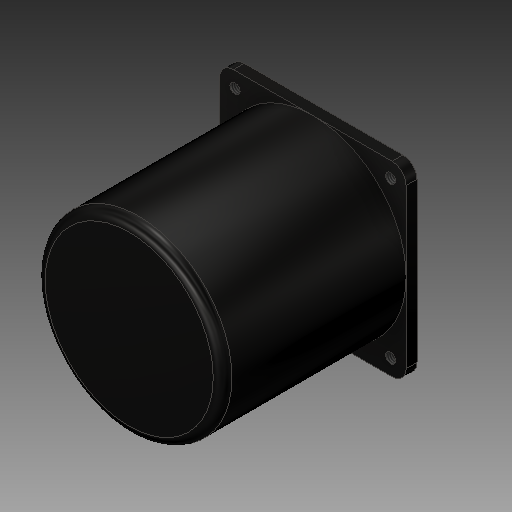
# Autodesk Inventor part: Moteur
Saved by Autodesk Inventor 2017 (Build 210142000, 142)
## iProperties
Company: FABLAB Frenchmakers
Part Number: Moteur
Project: 1400-PopCorn Machine
Material: Acier inoxydable
Catalog Web Link: http://www.frenchmakers.com/
Document SubType Name: Modeling
Designer: FABLAB Frenchmakers
Density: 8 g/cm^3
Appearance: Semi-poli
Stock Number: 1400-07-01
Mass: 1436.32 g
Surface Area: 193.93 cm^2
Volume: 179.539 cm^3
Author: Adrien MARY
Autodesk Inventor part; units mm, degrees
ref_plane "YZ Plane" through (0, 0, 0) normal (1, 0, 0) x (0, 1, 0)
ref_plane "XZ Plane" through (0, 0, 0) normal (0, 1, 0) x (-1, 0, 0)
ref_plane "XY Plane" through (0, 0, 0) normal (0, 0, 1) x (1, 0, 0)
sketch "Esquisse1" plane through (0, 0, 0) normal (0, 0, 1) x (1, 0, 0)
  line L0 (-25.5, -30) -> (25.5, -30)
  line L1 (30, -25.5) -> (30, 25.5)
  line L2 (25.5, 30) -> (-25.5, 30)
  line L3 (-30, 25.5) -> (-30, -25.5)
  line L4 (-30, -30) -> (30, 30) construction
  line L5 (30, -30) -> (-30, 30) construction
  arc A0 (-30, -25.5) -> (-25.5, -30) centre (-25.5, -25.5) ccw
  arc A1 (25.5, -30) -> (30, -25.5) centre (25.5, -25.5) ccw
  arc A2 (30, 25.5) -> (25.5, 30) centre (25.5, 25.5) ccw
  arc A3 (-25.5, 30) -> (-30, 25.5) centre (-25.5, 25.5) ccw
  point P0 (0, 0)
  dimension "d0" = 60
  dimension "d1" = 60
  dimension "d2" = 4.5
  constraints: 12 end point, 8 point on circle, 8 point on line, 8 tangent, 4 centre point, 3 equal radius, 2 midpoint, 2 parallel, 1 horizontal, 1 perpendicular
  measures "d0" distance of L5.end L4.end
  measures "d1" distance of L4.end L5.start
  measures "d2" radius of A0
extrude "Embase" add sketch "Esquisse1" along normal blind 3.5
sketch "Esquisse3" plane through (0, 0, 3.5) normal (0, 0, 1) x (1, 0, 0)
  point P0 (0, 0)
  point P1 (-25, -25)
  point P2 (-25, 25)
  point P3 (25, 25)
  point P4 (25, -25)
  dimension "Entraxe_moteur" = 50
  dimension "d8" = 50
  dimension "d9" = 25
  dimension "d10" = 25
  constraints: 2 horizontal alignment, 2 vertical alignment
  measures "Entraxe_moteur" distance of point (-25, 25) point (25, 25)
  measures "d8" distance of point (25, 25) point (25, -25)
  measures "d9" horizontal distance of point (25, 25) point (0, 0)
  measures "d10" horizontal distance of point (0, 0) point (25, 25)
hole "Perçage1" at (-25, -25, 3.5) at (-25, 25, 3.5) at (25, 25, 3.5) at (25, -25, 3.5) direction (0, 0, -1) diameter 3.242 end through all thread size "M4x0.7" class "6H" standard "ISO Metric profile"
sketch "Esquisse2" plane through (0, 0, 3.5) normal (0, 0, 1) x (1, 0, 0)
  circle A0 centre (0, 0) radius 30
  line L0 (-30, 25.5) -> (-30, -25.5) projected
  constraints: 1 centre point, 1 coincident, 1 tangent
extrude "Extrusion2" add sketch "Esquisse2" along normal blind 59
fillet "Congé1" radius 3 1 edges at (-30, 0, 62.5)
sketch "Esquisse4" plane through (0, 0, 0) normal (0, 0, -1) x (-1, 0, 0)
  circle A0 centre (0, 0) radius 3.5
  dimension "d19" = 7
  constraints: 1 centre point, 1 coincident
  measures "d19" diameter of A0
extrude "Extrusion3" add sketch "Esquisse4" along normal blind 19
sketch "Esquisse5" plane through (0, 0, -19) normal (0, 0, -1) x (-1, 0, 0)
  line L0 (-1.8028, -3) -> (1.8028, -3)
  circle A0 centre (0, 0) radius 3.5 projected
  dimension "d22" = 6.5
  constraints: 2 end point, 2 point on circle, 1 horizontal
extrude "Extrusion4" cut sketch "Esquisse5" against normal blind 15 contours L0 A0 picked at (0.3722, -3.1057)
sketch "Esquisse6" plane through (-1.8028, -3, -19) normal (0, -1, 0) x (1, 0, 0)
  line L0 (3.6056, 0) -> (0, 0) projected
  point P0 (1.8028, 19)
  point P1 (1.8028, 8)
  point P2 (1.8028, 0)
  dimension "d25" = 8
  constraints: 1 midpoint, 1 vertical alignment
  measures "d25" distance from line of L0 point (1.803, 8)
hole "Perçage2" at (0, -3, -11) direction (0, 1, 0) diameter 3.4 end through all clearance for "Vis à tête plate fraisée ISO 2009/7046" size "M3" standard "ISO"
equation "\"d8\" = Entraxe_moteur"
equation "\"d9\" = 0.5 * Entraxe_moteur"
equation "\"d10\" = 0.5 * Entraxe_moteur"
